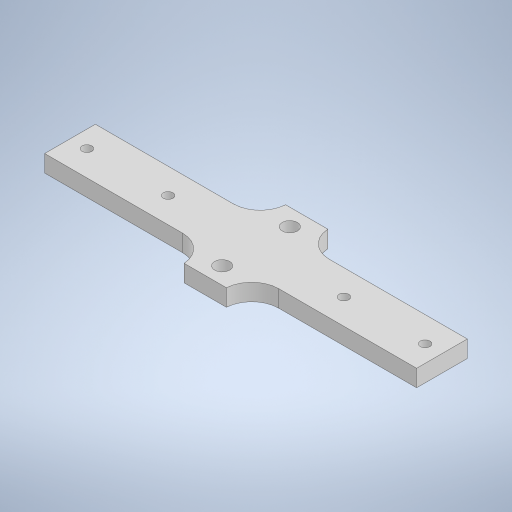
# Autodesk Inventor part: board2
Saved by Autodesk Inventor 2024 (Build 280153000, 153)
## iProperties
Created: 2024-10-06
Part Number: board2
Material: 一般
Document SubType Name: Modeling
Designer: 1412z
Density: 1 g/cm^3
Appearance: 既定
Author: 1412z
Autodesk Inventor part; units mm, degrees
ref_plane "YZ Plane" through (0, 0, 0) normal (1, 0, 0) x (0, 1, 0)
ref_plane "XZ Plane" through (0, 0, 0) normal (0, 1, 0) x (-1, 0, 0)
ref_plane "XY Plane" through (0, 0, 0) normal (0, 0, 1) x (1, 0, 0)
sketch "スケッチ1" plane through (0, 0, 0) normal (0, 1, 0) x (-1, 0, 0)
  line L0 (-55, -7.5) -> (55, -7.5)
  line L1 (55, -7.5) -> (55, 7.5)
  line L2 (55, 7.5) -> (-55, 7.5)
  line L3 (-55, 7.5) -> (-55, -7.5)
  line L4 (-55, -7.5) -> (55, 7.5) construction
  line L5 (55, -7.5) -> (-55, 7.5) construction
  point P0 (0, 0)
  dimension "d0" = 110
  dimension "d1" = 15
  constraints: 12 end point, 2 midpoint, 2 parallel, 1 horizontal, 1 perpendicular
  measures "d0" distance of L2.end L1.end
  measures "d1" distance of L1.end L0.end
extrude "押し出し1" add sketch "スケッチ1" along normal mid plane 5
sketch "スケッチ2" plane through (0, 2.5, 0) normal (0, 1, 0) x (1, 0, 0)
  circle A0 centre (50, 0) radius 1.45
  circle A1 centre (-50, 0) radius 1.45
  point P0 (0, 0)
  dimension "d4" = 2.9
  dimension "d5" = 2.9
  constraints: 2 centre point
  measures "d4" diameter of A0
  measures "d5" diameter of A1
extrude "押し出し2" cut sketch "スケッチ2" against normal blind 5
sketch "スケッチ3" plane through (0, 2.5, 0) normal (0, 1, 0) x (1, 0, 0)
  circle A0 centre (26, 0) radius 1.45
  circle A1 centre (-26, 0) radius 1.45
  point P0 (0, 0)
  dimension "d8" = 2.9
  dimension "d9" = 2.9
  constraints: 2 centre point
  measures "d8" diameter of A0
  measures "d9" diameter of A1
extrude "押し出し3" cut sketch "スケッチ3" against normal blind 5
sketch "スケッチ4" plane through (0, 2.5, 0) normal (0, 1, 0) x (1, 0, 0)
  line L0 (-6.25, 15) -> (6.25, 15)
  line L1 (6.25, 15) -> (6.25, -15)
  line L2 (6.25, -15) -> (-6.25, -15)
  line L3 (-6.25, -15) -> (-6.25, 15)
  line L4 (-6.25, 15) -> (6.25, -15) construction
  line L5 (6.25, 15) -> (-6.25, -15) construction
  point P0 (0, 0)
  dimension "d12" = 12.5
  dimension "d13" = 30
  constraints: 12 end point, 2 midpoint, 2 parallel, 1 horizontal, 1 perpendicular
  measures "d12" distance of L1.end L2.end
  measures "d13" distance of L0.end L1.end
extrude "押し出し4" add sketch "スケッチ4" against normal blind 5
fillet "フィレット1" radius 8 4 edges at (6.25, 0, 7.5) (-6.25, 0, 7.5) (-6.25, 0, -7.5) (6.25, 0, -7.5)
sketch "スケッチ5" plane through (0, 2.5, 0) normal (0, 1, 0) x (1, 0, 0)
  circle A0 centre (0, -10) radius 2.25
  circle A1 centre (0, 10) radius 2.25
  point P0 (0, 0)
  dimension "d17" = 4.5
  dimension "d18" = 4.5
  constraints: 2 centre point
  measures "d17" diameter of A0
  measures "d18" diameter of A1
extrude "押し出し5" cut sketch "スケッチ5" against normal blind 5
